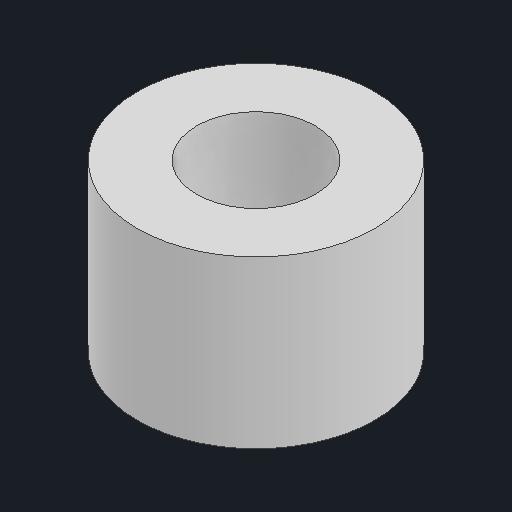
# Autodesk Inventor part: 라파hat간띄
Saved by Autodesk Inventor 2027.1 (Build 311270010, 270A)
## iProperties
Created: 2026-08-04
Part Number: 라파hat간띄
Material: 일반
Document SubType Name: Modeling
Designer: moieboy9999
Density: 1 g/cm^3
Appearance: 기본값
Mass: 0.0515418 g
Surface Area: 1.11919 cm^2
Volume: 0.0515418 cm^3
Author: moieboy9999
## iProperties of the stored document 라파hat간띄_3D 인쇄.ipt
Created: 2026-08-04
Part Number: 라파hat간띄_3D 인쇄
Material: 일반
Document SubType Name: Modeling
Designer: maker
Density: 1 g/cm^3
Appearance: 기본값
Author: maker
Autodesk Inventor part; units mm, degrees
ref_plane "YZ Plane" through (0, 0, 0) normal (1, 0, 0) x (0, 1, 0)
ref_plane "XZ Plane" through (0, 0, 0) normal (0, 1, 0) x (-1, 0, 0)
ref_plane "XY Plane" through (0, 0, 0) normal (0, 0, 1) x (1, 0, 0)
sketch "스케치1" plane through (0, 0, 0) normal (0, 1, 0) x (-1, 0, 0)
  circle A0 centre (0, 0) radius 1.25
  circle A1 centre (0, 0) radius 2.5
  dimension "d0" = 2.5
  dimension "d1" = 5
  constraints: 2 centre point, 2 coincident
  measures "d0" diameter of A0
  measures "d1" diameter of A1
extrude "돌출1" add sketch "스케치1" along normal blind 3.5
